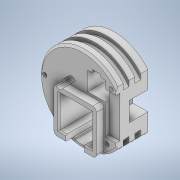
# Autodesk Inventor part: CameraBackSupport
Saved by Autodesk Inventor 2020 (Build 240168000, 168)
## iProperties
Created: 2019-08-28
Part Number: CameraBackSupport
Material: Generic
Document SubType Name: Modeling
Designer: rosbo
Density: 1 g/cm^3
Appearance: Default
Author: rosbo
Autodesk Inventor part; units mm, degrees
ref_plane "YZ Plane" through (0, 0, 0) normal (1, 0, 0) x (0, 1, 0)
sketch "Sketch1" plane through (0, 0, 0) normal (0, 0, 1) x (1, 0, 0)
  line L0 (-52.8422, 0) -> (52.8422, 0) projected
  line L1 (0, -52.8422) -> (0, 52.8422) projected
  circle A0 centre (0, 0) radius 37.7444
  dimension "d0" = 75.4888
  constraints: 1 centre point, 1 coincident
  measures "d0" diameter of A0
extrude "Extrusion1" add sketch "Sketch1" along normal blind 27.94
ref_plane "Work Plane1" through (0, 0, 21.59) normal (0, 0, 1) x (1, 0, 0)
sketch "Sketch2" plane through (0, 0, 21.59) normal (0, 0, 1) x (1, 0, 0)
  circle A0 centre (0, 0) radius 37.7444 projected
  line L0 (-52.8422, 0) -> (52.8422, 0) projected
  line L1 (0, -52.8422) -> (0, 52.8422) projected
  circle A1 centre (0, 0) radius 34.9504
  dimension "d32" = 2.794
  constraints: 1 centre point, 1 coincident
  measures "d32" radial gap between concentric circles of A0 A1
extrude "Extrusion2" cut sketch "Sketch2" against normal blind 4.953 contours L0 A1 L1 A0 | A0 L1 A1 L0 | L1 A1 L0 A0 | A0 L0 A1 L1
ref_plane "Work Plane2" through (0, 0, 6.35) normal (0, 0, -1) x (-1, 0, 0)
sketch "Sketch3" plane through (0, 0, 6.35) normal (0, 0, -1) x (-1, 0, 0)
  circle A0 centre (0, 0) radius 37.7444 projected
  circle A1 centre (0, 0) radius 34.9504 projected
extrude "Extrusion3" cut sketch "Sketch3" against normal blind 4.953
chamfer "Chamfer1" distance 1.778 angle 45 1 edges at (-37.7444, 0, 27.94)
sketch "Sketch5" plane through (0, 0, 27.94) normal (0, 0, 1) x (1, 0, 0)
  circle A0 centre (-33.02, 2.54) radius 1.778
  circle A1 centre (21.59, -22.86) radius 1.778
  circle A2 centre (-21.59, -22.86) radius 1.778
  line L0 (-52.8422, 0) -> (52.8422, 0) projected
  line L1 (0, -52.8422) -> (0, 52.8422) projected
  circle A3 centre (0, 0) radius 31.75
  circle A4 centre (0, 0) radius 34.9504 projected
  circle A5 centre (25.273, 20.828) radius 1.778
  dimension "d24" = 21.59
  dimension "d25" = 22.86
  dimension "d26" = 3.556
  dimension "d27" = 3.556
  dimension "d28" = 3.556
  dimension "d93" = 63.5
  dimension "d165" = 20.828
  dimension "d166" = 25.273
  dimension "d167" = 3.556
  dimension "d168" = 33.02
  dimension "d169" = 2.54
  constraints: 5 centre point, 1 coincident, 1 symmetric about line
  measures "d24" distance from line of A1.centre L1
  measures "d25" distance from line of A1.centre L0
  measures "d26" diameter of A1
  measures "d27" diameter of A2
  measures "d28" diameter of A0
  measures "d93" diameter of A3
  measures "d165" distance from line of A5.centre L0
  measures "d166" distance from line of A5.centre L1
  measures "d167" diameter of A5
  measures "d168" distance from line of A0.centre L1
  measures "d169" distance from line of A0.centre L0
extrude "Extrusion5" cut sketch "Sketch5" against normal through all contours A0 A3 | A3 A0 | A5 A3 | A3 A5 | A3 A2 | A2 A3 | A3 A1 | A1 A3
sketch "Sketch7" plane through (0, 0, 27.94) normal (0, 0, 1) x (1, 0, 0)
  line L0 (14.9225, -28.448) -> (-14.9225, -28.448) projected
  line L1 (14.9225, -34.163) -> (14.9225, -28.448) projected
  line L2 (-14.9225, -34.163) -> (14.9225, -34.163) projected
  line L3 (-14.9225, -28.448) -> (-14.9225, -34.163) projected
  circle A0 centre (-9.8806, -30.607) radius 1.778 projected
  circle A1 centre (9.8806, -30.607) radius 1.778 projected
  line L4 (-14.224, 1.143) -> (14.224, 1.143)
  line L5 (14.224, 1.143) -> (14.224, -27.305)
  line L6 (14.224, -27.305) -> (-14.224, -27.305)
  line L7 (-14.224, -27.305) -> (-14.224, 1.143)
  line L8 (-52.8422, 0) -> (52.8422, 0) projected
  line L9 (0, -52.8422) -> (0, 52.8422) projected
  line L10 (-18.669, 6.223) -> (18.669, 6.223)
  line L11 (18.669, 6.223) -> (18.669, -32.385)
  line L12 (18.669, -32.385) -> (-18.669, -32.385)
  line L13 (-18.669, -32.385) -> (-18.669, 6.223)
  point P0 (0, 0)
  dimension "d38" = 6.858
  dimension "d39" = 28.448
  dimension "d40" = 28.448
  dimension "d41" = 4.445
  dimension "d42" = 5.08
  dimension "d43" = 5.08
  constraints: 16 end point, 4 parallel, 2 horizontal, 2 perpendicular, 2 other
  measures "d38" distance between parallel lines of L6 L2
  measures "d39" distance between parallel lines of L4 L6
  measures "d40" distance between parallel lines of L5 L7
  measures "d41" distance between parallel lines of L11 L5
  measures "d42" distance between parallel lines of L10 L4
  measures "d43" distance between parallel lines of L6 L12
extrude "Extrusion7" add sketch "Sketch7" along normal blind 6.477 contours A1 | L1 L12 L9 L0 | L0 L9 L6 L5 L8 L11 L12 L1 | A0 | L9 L12 L3 L0 | L0 L3 L12 L13 L8 L7 L6 L9 | L8 L5 L4 L9 L10 L11 | L8 L13 L10 L9 L4 L7
sketch "Sketch8" plane through (0, 0, 34.417) normal (0, 0, 1) x (1, 0, 0)
  line L0 (18.669, -32.385) -> (18.669, 6.223) projected
  line L1 (18.669, 6.223) -> (-18.669, 6.223) projected
  line L2 (-18.669, 6.223) -> (-18.669, -32.385) projected
  line L3 (-18.669, -32.385) -> (18.669, -32.385) projected
  line L4 (-14.224, 1.143) -> (14.224, 1.143) projected
  line L5 (14.224, 1.143) -> (14.224, -27.305) projected
  line L6 (14.224, -27.305) -> (-14.224, -27.305) projected
  line L7 (-14.224, -27.305) -> (-14.224, 1.143) projected
  line L8 (14.224, -27.305) -> (-14.224, -27.305) projected
  line L9 (-8.0645, -27.305) -> (8.0645, -27.305)
  line L10 (8.0645, -27.305) -> (8.0645, -32.385)
  line L11 (8.0645, -32.385) -> (-8.0645, -32.385)
  line L12 (-8.0645, -32.385) -> (-8.0645, -27.305)
  line L13 (52.8422, 0) -> (-52.8422, 0)
  line L14 (0, -52.8422) -> (0, 52.8422)
  line L15 (0, -52.8422) -> (0, 52.8422)
  point P0 (0, 0)
  dimension "d46" = 16.129
  constraints: 14 end point, 2 horizontal, 2 parallel, 2 point on line, 2 vertical, 1 perpendicular, 7 other
  measures "d46" distance between parallel lines of L10 L12
extrude "Extrusion8" cut sketch "Sketch8" against normal up to surface (6.477 mm away) contours L3 L14 L6 L10 | L3 L12 L6 L14
sketch "Sketch11" plane through (0, 0, 27.94) normal (0, 0, 1) x (1, 0, 0)
  line L0 (8.0645, -27.305) -> (8.0645, -32.385) projected
  line L1 (8.0645, -32.385) -> (18.669, -32.385) projected
  line L2 (18.669, -32.385) -> (18.669, 6.223) projected
  line L3 (18.669, 6.223) -> (-18.669, 6.223) projected
  line L4 (-18.669, 6.223) -> (-18.669, -32.385) projected
  line L5 (-18.669, -32.385) -> (-8.0645, -32.385) projected
  line L6 (-8.0645, -32.385) -> (-8.0645, -27.305) projected
  line L7 (-8.0645, -27.305) -> (-14.224, -27.305) projected
  line L8 (-14.224, -27.305) -> (-14.224, 1.143) projected
  line L9 (-14.224, 1.143) -> (14.224, 1.143) projected
  line L10 (14.224, 1.143) -> (14.224, -27.305) projected
  line L11 (14.224, -27.305) -> (8.0645, -27.305) projected
  line L12 (-8.0645, -32.385) -> (8.0645, -32.385)
  line L13 (8.0645, -32.385) -> (8.0645, -16.256)
  line L14 (8.0645, -16.256) -> (-8.0645, -16.256)
  line L15 (-8.0645, -16.256) -> (-8.0645, -32.385)
  point P0 (0, 0)
  dimension "d64" = 16.129
  constraints: 8 end point, 2 parallel, 1 horizontal, 1 perpendicular
  measures "d64" distance of L13.end L12.end
extrude "Extrusion11" cut sketch "Sketch11" against normal up to surface (27.94 mm away) contours L0 L12 L6 L15 L14 L13
fillet "Fillet3" radius 3.175 2 edges at (18.669, 6.223, 31.1785) (-18.669, 6.223, 31.1785)
sketch "Sketch12" plane through (0, 0, 27.94) normal (0, 0, 1) x (1, 0, 0)
  line L0 (-8.0645, -27.305) -> (-8.0645, -16.256) projected
  line L1 (-8.0645, -16.256) -> (8.0645, -16.256) projected
  line L2 (8.0645, -16.256) -> (8.0645, -27.305) projected
  line L3 (8.0645, -27.305) -> (14.224, -27.305) projected
  line L4 (14.224, -27.305) -> (14.224, 1.143) projected
  line L5 (14.224, 1.143) -> (-14.224, 1.143) projected
  line L6 (-14.224, 1.143) -> (-14.224, -27.305) projected
  line L7 (-14.224, -27.305) -> (-8.0645, -27.305) projected
  point P0 (0, 0)
extrude "Extrusion12" cut sketch "Sketch12" against normal blind 22.86
fillet "Fillet5" radius 3.175 2 edges at (18.669, -32.385, 31.1785) (-18.669, -32.385, 31.1785)
sketch "Sketch13" plane through (0, 0, 27.94) normal (0, 0, 1) x (1, 0, 0)
  line L0 (8.0645, -32.385) -> (-8.0645, -32.385) projected
  line L1 (-8.0645, -32.385) -> (-15.494, -32.385) projected
  arc A0 (-15.6543, -32.381) -> (-15.494, -32.385) centre (-15.494, -29.21) ccw projected
  arc A1 (-15.6543, -32.381) -> (15.6543, -32.381) centre (0, 0) ccw projected
  arc A2 (-18.669, -29.21) -> (-15.494, -32.385) centre (-15.494, -29.21) ccw projected
  line L2 (-15.494, -32.385) -> (-8.0645, -32.385) projected
  line L3 (-8.0645, -32.385) -> (-8.0645, -27.305) projected
  line L4 (-8.0645, -27.305) -> (-14.224, -27.305) projected
  line L5 (-14.224, -27.305) -> (-14.224, 1.143) projected
  line L6 (-14.224, 1.143) -> (14.224, 1.143) projected
  line L7 (14.224, 1.143) -> (14.224, -27.305) projected
  line L8 (14.224, -27.305) -> (8.0645, -27.305) projected
  line L9 (8.0645, -27.305) -> (8.0645, -32.385) projected
  line L10 (18.669, -29.21) -> (18.669, 3.048) projected
  arc A3 (18.669, 3.048) -> (15.494, 6.223) centre (15.494, 3.048) ccw projected
  line L11 (15.494, 6.223) -> (-15.494, 6.223) projected
  arc A4 (-15.494, 6.223) -> (-18.669, 3.048) centre (-15.494, 3.048) ccw projected
  line L12 (-18.669, 3.048) -> (-18.669, -29.21) projected
  circle A5 centre (0, 0) radius 34.9504 projected
  circle A6 centre (0, 0) radius 34.9504 projected
  circle A7 centre (0, 0) radius 34.9504 projected
  line L13 (-6.35, -32.385) -> (-6.35, -33.655)
  line L14 (6.35, -33.655) -> (6.35, -32.385)
  line L15 (0, -52.8422) -> (0, 52.8422) projected
  arc A8 (-6.35, -33.655) -> (6.35, -33.655) centre (0, 0) ccw
  arc A9 (-18.669, -28.7132) -> (-18.6335, -28.7363) centre (0, 0) ccw
  line L16 (8.0645, -32.385) -> (15.494, -32.385) projected
  line L17 (18.669, 3.048) -> (18.669, -29.21) projected
  arc A10 (18.0294, -31.1211) -> (-18.0294, -31.1211) centre (0, 0) ccw projected
  arc A11 (-18.669, -29.21) -> (-18.0294, -31.1211) centre (-15.494, -29.21) ccw projected
  line L18 (-18.669, -29.21) -> (-18.669, 3.048) projected
  arc A12 (-15.494, 6.223) -> (-18.669, 3.048) centre (-15.494, 3.048) ccw projected
  line L19 (-15.494, 6.223) -> (15.494, 6.223) projected
  arc A13 (18.669, 3.048) -> (15.494, 6.223) centre (15.494, 3.048) ccw projected
  line L20 (15.494, -32.385) -> (8.0645, -32.385) projected
  arc A14 (15.494, -32.385) -> (18.669, -29.21) centre (15.494, -29.21) ccw projected
  arc A15 (18.0294, -31.1211) -> (18.669, -29.21) centre (15.494, -29.21) ccw projected
  arc A16 (15.494, -32.385) -> (15.6543, -32.381) centre (15.494, -29.21) ccw projected
  dimension "d79" = 12.7
  constraints: 5 point on circle, 4 end point, 3 point on line, 2 centre point, 1 coincident, 1 perpendicular, 1 vertical, 1 other
  measures "d79" distance between parallel lines of L14 L13
extrude "Extrusion13" cut sketch "Sketch13" against normal through all contours L14 A8 L15 L0 | L15 A8 L13 L0
chamfer "Chamfer4" distance 1.016 angle 45 5 edges at (-14.224, -13.081, 34.417) (0, 1.143, 34.417) (14.224, -13.081, 34.417) (11.1442, -27.305, 34.417) (-11.1443, -27.305, 34.417)
sketch "Sketch19" plane through (0, 0, 0) normal (0, 0, -1) x (-1, 0, 0)
  line L0 (-19.1897, 31.0124) -> (19.1897, 31.0124)
  line L1 (19.1897, 31.0124) -> (19.1897, -4.4714)
  line L2 (19.1897, -4.4714) -> (-19.1897, -4.4714)
  line L3 (-19.1897, -4.4714) -> (-19.1897, 31.0124)
  line L4 (52.8422, 0) -> (-52.8422, 0) projected
  line L5 (0, -52.8422) -> (0, 52.8422) projected
  circle A0 centre (-14.9987, 27.0754) radius 1.651
  circle A1 centre (14.9987, 27.0754) radius 1.651
  circle A2 centre (-14.9987, 15.0866) radius 1.651
  circle A3 centre (14.9987, 15.0866) radius 1.651
  line L6 (-9.271, 31.0124) -> (9.271, 31.0124)
  line L7 (9.271, 31.0124) -> (9.271, 11.7084)
  line L8 (9.271, 11.7084) -> (-9.271, 11.7084)
  line L9 (-9.271, 11.7084) -> (-9.271, 31.0124)
  line L10 (-18.034, 3.6566) -> (18.034, 3.6566)
  line L11 (18.034, 3.6566) -> (18.034, -3.0744)
  line L12 (18.034, -3.0744) -> (-18.034, -3.0744)
  line L13 (-18.034, -3.0744) -> (-18.034, 3.6566)
  circle A4 centre (0, 0) radius 34.9504 projected
  circle A5 centre (0, 0) radius 37.7444 projected
  circle A6 centre (33.02, 2.54) radius 1.778 projected
  circle A7 centre (21.59, -22.86) radius 1.778 projected
  circle A8 centre (-21.59, -22.86) radius 1.778 projected
  line L14 (6.35, -32.385) -> (6.35, -33.655) projected
  arc A9 (-6.35, -33.655) -> (6.35, -33.655) centre (0, 0) ccw projected
  line L15 (-6.35, -33.655) -> (-6.35, -32.385) projected
  line L16 (-6.35, -32.385) -> (-8.0645, -32.385) projected
  line L17 (-8.0645, -32.385) -> (-8.0645, -16.256) projected
  line L18 (-8.0645, -16.256) -> (8.0645, -16.256) projected
  line L19 (8.0645, -16.256) -> (8.0645, -32.385) projected
  line L20 (8.0645, -32.385) -> (6.35, -32.385) projected
  dimension "d112" = 38.3794
  dimension "d113" = 35.4838
  dimension "d114" = 29.9974
  dimension "d115" = 3.302
  dimension "d116" = 3.302
  dimension "d117" = 3.937
  dimension "d118" = 3.302
  dimension "d119" = 3.302
  dimension "d120" = 29.9974
  dimension "d121" = 11.9888
  dimension "d122" = 18.542
  dimension "d123" = 19.304
  dimension "d124" = 36.068
  dimension "d125" = 6.731
  dimension "d126" = 1.397
  constraints: 24 end point, 6 parallel, 4 centre point, 3 horizontal, 3 perpendicular, 2 symmetric about line, 1 point on line, 3 other
  measures "d112" distance of L1.end L2.end
  measures "d113" distance of L0.end L1.end
  measures "d114" distance of A1.centre A0.centre
  measures "d115" diameter of A1
  measures "d116" diameter of A0
  measures "d117" distance from line of A0.centre L0
  measures "d118" diameter of A3
  measures "d119" diameter of A2
  measures "d120" distance of A3.centre A2.centre
  measures "d121" distance of A2.centre A0.centre
  measures "d122" distance of L7.end L8.end
  measures "d123" distance of L6.end L7.end
  measures "d124" distance of L11.end L12.end
  measures "d125" distance of L10.end L11.end
  measures "d126" distance between parallel lines of L12 L2
sketch "Sketch21" plane through (0, 0, 0) normal (0, 0, -1) x (-1, 0, 0)
  circle A0 centre (0, 0) radius 34.9504 projected
  line L0 (52.8422, 0) -> (-52.8422, 0) projected
  line L1 (0, -52.8422) -> (0, 52.8422) projected
  circle A1 centre (0, 0) radius 31.7754
  line L2 (-29.3624, 8.4074) -> (-16.0782, 8.4074)
  line L3 (-16.0782, 8.4074) -> (-16.0782, -8.4074)
  line L4 (-16.0782, -8.4074) -> (-29.3624, -8.4074)
  line L5 (-29.3624, -8.4074) -> (-29.3624, 8.4074)
  line L6 (-30.7115, -18.669) -> (-30.7115, 18.669)
  dimension "d133" = 63.5508
  dimension "d134" = 13.2842
  dimension "d135" = 16.8148
  dimension "d136" = 37.338
  dimension "d150" = 16.0782
  constraints: 10 end point, 2 parallel, 1 centre point, 1 coincident, 1 horizontal, 1 perpendicular, 1 symmetric about line, 1 vertical, 1 other
  measures "d133" diameter of A1
  measures "d134" distance of L3.end L4.end
  measures "d135" distance of L2.end L3.end
  measures "d136" distance of L6.start L6.end
  measures "d150" distance between parallel lines of L1 L3
extrude "Extrusion19" cut sketch "Sketch21" against normal blind 16.256 contours L3 L4 L5 L0 | L0 L5 L2 L3
sketch "Sketch22" plane through (0, 0, 0) normal (0, 0, -1) x (-1, 0, 0)
  line L0 (-29.3624, -8.4074) -> (-29.3624, 8.4074) projected
  line L1 (-16.0782, 8.4074) -> (-16.0782, -8.4074) projected
  line L2 (-16.0782, -8.4074) -> (-29.3624, -8.4074) projected
  line L3 (-29.3624, -8.4074) -> (-29.3624, 8.4074) projected
  line L4 (-29.3624, 8.4074) -> (-16.0782, 8.4074) projected
  circle A0 centre (0, 0) radius 37.7444 projected
  circle A1 centre (33.02, 2.54) radius 1.778 projected
  circle A2 centre (21.59, -22.86) radius 1.778 projected
  circle A3 centre (-21.59, -22.86) radius 1.778 projected
  line L5 (6.35, -32.385) -> (6.35, -33.655) projected
  arc A4 (-6.35, -33.655) -> (6.35, -33.655) centre (0, 0) ccw projected
  line L6 (-6.35, -33.655) -> (-6.35, -32.385) projected
  line L7 (-6.35, -32.385) -> (-8.0645, -32.385) projected
  line L8 (-8.0645, -32.385) -> (-8.0645, -16.256) projected
  line L9 (-8.0645, -16.256) -> (8.0645, -16.256) projected
  line L10 (8.0645, -16.256) -> (8.0645, -32.385) projected
  line L11 (8.0645, -32.385) -> (6.35, -32.385) projected
  line L12 (-29.3624, -23.7169) -> (-29.3624, 23.7169)
  constraints: 2 end point, 2 point on circle, 1 collinear, 1 vertical
extrude "Extrusion20" cut sketch "Sketch22" against normal through all contours L12 A0 L0
sketch "Sketch23" plane through (29.3624, 8.4074, 0) normal (1, 0, 0) x (0, 0, -1)
  line L0 (0, 0) -> (-16.256, 0) projected
  line L1 (0, 15.3095) -> (0, 0) projected
  line L2 (-6.35, 15.3095) -> (0, 15.3095) projected
  line L3 (-6.35, 10.5499) -> (-6.35, 15.3095) projected
  line L4 (-11.303, 10.5499) -> (-6.35, 10.5499) projected
  line L5 (-11.303, 15.3095) -> (-11.303, 10.5499) projected
  line L6 (-16.637, 15.3095) -> (-11.303, 15.3095) projected
  line L7 (-16.637, 10.5499) -> (-16.637, 15.3095) projected
  line L8 (-21.59, 10.5499) -> (-16.637, 10.5499) projected
  line L9 (-21.59, 15.3095) -> (-21.59, 10.5499) projected
  line L10 (-26.162, 15.3095) -> (-21.59, 15.3095) projected
  line L11 (-27.94, -29.1783) -> (-27.94, 12.3635) projected
  line L12 (-21.59, -32.1243) -> (-26.162, -32.1243) projected
  line L13 (-21.59, -27.3647) -> (-21.59, -32.1243) projected
  line L14 (-16.637, -27.3647) -> (-21.59, -27.3647) projected
  line L15 (-16.637, -32.1243) -> (-16.637, -27.3647) projected
  line L16 (-11.303, -32.1243) -> (-16.637, -32.1243) projected
  line L17 (-11.303, -27.3647) -> (-11.303, -32.1243) projected
  line L18 (-6.35, -27.3647) -> (-11.303, -27.3647) projected
  line L19 (-6.35, -32.1243) -> (-6.35, -27.3647) projected
  line L20 (0, -32.1243) -> (-6.35, -32.1243) projected
  line L21 (0, -16.8148) -> (0, -32.1243) projected
  line L22 (0, -16.8148) -> (-16.256, -16.8148) projected
  line L23 (-16.256, -16.8148) -> (-16.256, 0) projected
  line L24 (0, -61.2496) -> (0, 44.4348) projected
  line L25 (6.8834, -8.4074) -> (-41.3004, -8.4074) projected
  line L26 (-31.2674, 9.6901) -> (-24.5364, 9.6901)
  line L27 (-24.5364, 9.6901) -> (-24.5364, -26.5049)
  line L28 (-24.5364, -26.5049) -> (-31.2674, -26.5049)
  line L29 (-31.2674, -26.5049) -> (-31.2674, 9.6901)
  point P0 (0, -8.4074)
  dimension "d141" = 6.731
  dimension "d142" = 36.195
  dimension "d143" = 8.2804
  constraints: 8 end point, 2 parallel, 1 horizontal, 1 perpendicular, 3 other
  measures "d141" distance of L27.end L28.end
  measures "d142" distance of L26.end L27.end
  measures "d143" distance between parallel lines of L27 L23
extrude "Extrusion21" cut sketch "Sketch23" against normal blind 9.1694 contours L28 L29 L25 L11 | L11 L25 L27 L28 | L25 L29 L26 L11 | L11 L26 L27 L25
sketch "Sketch28" plane through (0, 0, 27.94) normal (0, 0, 1) x (1, 0, 0)
  line L0 (-52.8422, 0) -> (52.8422, 0) projected
  line L1 (0, -52.8422) -> (0, 52.8422) projected
  line L2 (-15.494, 6.223) -> (15.494, 6.223) projected
  line L3 (4.4768, 24.9174) -> (20.193, 24.9174)
  line L4 (20.193, 24.9174) -> (20.193, 8.4074)
  line L5 (4.4768, 8.4074) -> (4.4768, 24.9174)
  line L6 (20.193, -18.0975) -> (20.193, 18.0975) projected
  line L7 (4.4768, 8.4074) -> (20.193, 8.4074)
  point P0 (0, 0)
  point P1 (0.362, 6.223)
  point P2 (16.0782, 6.223)
  dimension "d170" = 15.7163
  dimension "d187" = 2.1844
  dimension "d188" = 0
  dimension "d189" = 16.51
  constraints: 8 end point, 2 horizontal, 2 point on line, 1 parallel, 1 perpendicular
  measures "d170" distance between parallel lines of L4 L5
  measures "d187" distance between parallel lines of L7 L2
  measures "d188" distance between parallel lines of L6 L4
  measures "d189" distance between parallel lines of L7 L3
extrude "Extrusion26" cut sketch "Sketch28" against normal through all
sketch "Sketch29" plane through (0, 0, 27.94) normal (0, 0, 1) x (1, 0, 0)
  line L0 (20.193, 24.9174) -> (20.193, 18.0975) projected
  arc A0 (18.669, 3.048) -> (15.494, 6.223) centre (15.494, 3.048) ccw projected
  line L1 (18.669, 3.048) -> (18.669, -29.21) projected
  arc A1 (18.0294, -31.1211) -> (18.669, -29.21) centre (15.494, -29.21) ccw projected
  arc A2 (18.0294, -31.1211) -> (29.3624, -20.7709) centre (0, 0) ccw projected
  line L2 (29.3624, -20.7709) -> (29.3624, -18.0975) projected
  line L3 (29.3624, -18.0975) -> (20.193, -18.0975) projected
  line L4 (20.193, -18.0975) -> (20.193, 8.4074) projected
  line L5 (20.193, 18.0975) -> (29.3624, 18.0975) projected
  line L6 (29.3624, 18.0975) -> (29.3624, 20.7709) projected
  arc A3 (29.3624, 20.7709) -> (-18.0294, -31.1211) centre (0, 0) ccw projected
  arc A4 (-18.669, -29.21) -> (-18.0294, -31.1211) centre (-15.494, -29.21) ccw projected
  line L7 (-18.669, -29.21) -> (-18.669, 3.048) projected
  arc A5 (-15.494, 6.223) -> (-18.669, 3.048) centre (-15.494, 3.048) ccw projected
  line L8 (20.193, 8.4074) -> (4.4768, 8.4074) projected
  line L9 (4.4768, 8.4074) -> (4.4768, 24.9174) projected
  line L10 (4.4768, 24.9174) -> (20.193, 24.9174) projected
  circle A6 centre (21.59, -22.86) radius 1.778 projected
  circle A7 centre (-33.02, 2.54) radius 1.778 projected
  circle A8 centre (-21.59, -22.86) radius 1.778 projected
  circle A9 centre (25.273, 20.828) radius 1.778 projected
  line L11 (4.4768, 24.9174) -> (20.193, 24.9174) projected
  line L12 (8.5281, 24.9174) -> (16.1417, 24.9174)
  line L13 (16.1417, 24.9174) -> (16.1417, 27.4574)
  line L14 (16.1417, 27.4574) -> (8.5281, 27.4574)
  line L15 (8.5281, 27.4574) -> (8.5281, 24.9174)
  line L16 (0, -55.4557) -> (0, 68.5233) projected
  line L17 (-15.494, 6.223) -> (15.494, 6.223) projected
  dimension "d174" = 2.54
  dimension "d185" = 4.0513
  dimension "d186" = 4.0513
  constraints: 8 end point, 2 perpendicular, 1 collinear, 1 horizontal, 1 parallel
  measures "d174" distance of L13.end L12.end
  measures "d185" distance between parallel lines of L9 L15
  measures "d186" distance between parallel lines of L0 L13
extrude "Extrusion27" cut sketch "Sketch29" against normal blind 6.35 contours L10 L15 L14 L13
sketch "Sketch33" plane through (0, 0, 0) normal (0, 0, -1) x (-1, 0, 0)
  line L0 (6.0848, 11.1501) -> (11.9263, 5.3173) projected
  arc A0 (11.9263, 5.3173) -> (16.4164, 5.3206) centre (14.1697, 7.564) ccw projected
  line L1 (16.4164, 5.3206) -> (17.7625, 6.6686) projected
  line L2 (17.7625, 6.6686) -> (11.921, 12.5015) projected
  arc A1 (11.921, 12.5015) -> (7.4309, 12.4982) centre (9.6776, 10.2547) ccw projected
  line L3 (7.4309, 12.4982) -> (6.0848, 11.1501) projected
  point P0 (0, 0)
extrude "Extrusion30" cut sketch "Sketch33" against normal through all
sketch "Sketch31" plane through (0, 0, 0) normal (0, 0, -1) x (-1, 0, 0)
  line L0 (18.669, 3.048) -> (18.669, -29.21) projected
  line L1 (15.24, -28.321) -> (8.0645, -28.321) projected
  line L2 (15.24, 2.159) -> (15.24, -28.321) projected
  line L3 (-15.24, 2.159) -> (15.24, 2.159) projected
  line L4 (-15.24, -28.321) -> (-15.24, 2.159) projected
  line L5 (-8.0645, -28.321) -> (-15.24, -28.321) projected
  line L6 (-8.0645, -28.321) -> (-8.0645, -32.385) projected
  line L7 (-8.0645, -32.385) -> (-15.494, -32.385) projected
  arc A0 (-18.669, -29.21) -> (-15.494, -32.385) centre (-15.494, -29.21) ccw projected
  line L8 (-18.669, -29.21) -> (-18.669, 3.048) projected
  arc A1 (-15.494, 6.223) -> (-18.669, 3.048) centre (-15.494, 3.048) ccw projected
  line L9 (-15.494, 6.223) -> (15.494, 6.223) projected
  arc A2 (18.669, 3.048) -> (15.494, 6.223) centre (15.494, 3.048) ccw projected
  line L10 (18.669, 3.048) -> (18.669, -29.21) projected
  arc A3 (15.494, -32.385) -> (18.669, -29.21) centre (15.494, -29.21) ccw projected
  line L11 (15.494, -32.385) -> (8.0645, -32.385) projected
  line L12 (8.0645, -32.385) -> (8.0645, -28.321) projected
  line L13 (9.0145, 20.8534) -> (28.3185, 20.8534)
  line L14 (28.3185, 20.8534) -> (28.3185, 8.4074)
  line L15 (28.3185, 8.4074) -> (9.0145, 8.4074)
  line L16 (9.0145, 8.4074) -> (9.0145, 20.8534)
  line L17 (-4.4768, 8.4074) -> (-16.0782, 8.4074) projected
  point P0 (0, 0)
  dimension "d190" = 19.304
  dimension "d191" = 12.446
  constraints: 8 end point, 2 parallel, 1 collinear, 1 horizontal, 1 perpendicular
  measures "d190" distance of L14.end L15.end
  measures "d191" distance of L13.end L14.end
sketch "Sketch25" plane through (0, 0, 27.94) normal (0, 0, 1) x (1, 0, 0)
  line L0 (-52.8422, 0) -> (52.8422, 0) projected
  line L1 (0, -52.8422) -> (0, 52.8422) projected
  line L2 (-19.939, 21.8694) -> (19.939, 21.8694)
  line L3 (19.939, 21.8694) -> (19.939, 8.4074)
  line L4 (19.939, 8.4074) -> (-19.939, 8.4074)
  line L5 (-19.939, 8.4074) -> (-19.939, 21.8694)
  line L6 (-14.224, 1.143) -> (14.224, 1.143) projected
  line L7 (15.494, 6.223) -> (-15.494, 6.223) projected
  point P0 (0, 0)
  dimension "d153" = 39.878
  dimension "d154" = 13.462
  dimension "d164" = 2.1844
  constraints: 8 end point, 1 horizontal, 1 parallel, 1 perpendicular, 1 other
  measures "d153" distance of L3.end L4.end
  measures "d154" distance between parallel lines of L4 L2
  measures "d164" distance between parallel lines of L4 L7
sketch "Sketch26" plane through (0, 0, 27.94) normal (0, 0, 1) x (1, 0, 0)
  circle A0 centre (-33.02, 2.54) radius 1.778 projected
  circle A1 centre (-21.59, -22.86) radius 1.778 projected
  circle A2 centre (21.59, -22.86) radius 1.778 projected
  line L0 (-15.494, 6.223) -> (15.494, 6.223) projected
  arc A3 (18.669, 3.048) -> (15.494, 6.223) centre (15.494, 3.048) ccw projected
  line L1 (18.669, 3.048) -> (18.669, -29.21) projected
  arc A4 (18.0294, -31.1211) -> (18.669, -29.21) centre (15.494, -29.21) ccw projected
  arc A5 (18.0294, -31.1211) -> (29.3624, -20.7709) centre (0, 0) ccw projected
  line L2 (29.3624, -20.7709) -> (29.3624, -18.0975) projected
  line L3 (29.3624, -18.0975) -> (20.193, -18.0975) projected
  line L4 (20.193, -18.0975) -> (20.193, 18.0975) projected
  line L5 (20.193, 18.0975) -> (29.3624, 18.0975) projected
  line L6 (29.3624, 18.0975) -> (29.3624, 20.7709) projected
  arc A6 (29.3624, 20.7709) -> (-18.0294, -31.1211) centre (0, 0) ccw projected
  arc A7 (-18.669, -29.21) -> (-18.0294, -31.1211) centre (-15.494, -29.21) ccw projected
  line L7 (-18.669, -29.21) -> (-18.669, 3.048) projected
  arc A8 (-15.494, 6.223) -> (-18.669, 3.048) centre (-15.494, 3.048) ccw projected
  line L8 (20.193, 18.0975) -> (29.3624, 18.0975) projected
  line L9 (20.193, 18.0975) -> (19.8755, 18.0975)
  line L10 (19.939, 8.4074) -> (20.193, 8.4074)
  circle A9 centre (25.273, 20.066) radius 1.778 projected
  constraints: 4 end point, 1 horizontal, 1 point on line
sketch "Sketch27" plane through (0, 0, 17.78) normal (0, 0, 1) x (1, 0, 0)
  line L0 (-19.939, 8.4074) -> (-19.939, 21.8694) projected
  line L1 (19.939, 8.4074) -> (-19.939, 8.4074) projected
  line L2 (19.939, 21.8694) -> (19.939, 8.4074) projected
  line L3 (-19.939, 21.8694) -> (19.939, 21.8694) projected
  line L4 (-19.939, 13.1064) -> (-8.5217, 13.1064)
  line L5 (-8.5217, 13.1064) -> (-8.5217, 27.0764)
  line L6 (-8.5217, 27.0764) -> (8.5217, 27.0764)
  line L7 (8.5217, 27.0764) -> (8.5217, 13.1064)
  line L8 (8.5217, 13.1064) -> (19.939, 13.1064)
  line L9 (-52.8422, 0) -> (52.8422, 0) projected
  line L10 (0, -52.8422) -> (0, 52.8422) projected
  point P0 (0, 0)
  point P1 (-8.5217, 21.8694)
  point P2 (8.5217, 21.8694)
  dimension "d159" = 17.0434
  dimension "d160" = 13.97
  dimension "d161" = 4.699
  constraints: 10 end point, 4 point on line, 3 perpendicular, 1 horizontal, 1 other
  measures "d159" distance between parallel lines of L7 L5
  measures "d160" distance between parallel lines of L8 L6
  measures "d161" distance between parallel lines of L1 L8
body "Solid1"
